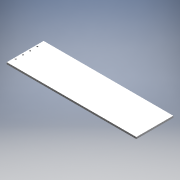
# Autodesk Inventor part: AluminumPlateForWinch
Saved by Autodesk Inventor 2018.2 (Build 222227000, 227)
## iProperties
Created: 2018-01-31
Part Number: AluminumPlateForWinch
Material: Aluminum 6061
Document SubType Name: Modeling
Designer: steele
Mass: 1020.4 g
Surface Area: 1264.92 cm^2
Volume: 377.927 cm^3
Density: 2.7 g/cm^3
Appearance: Aluminum - Flat
Author: steele
Autodesk Inventor part; units mm, degrees
ref_plane "YZ Plane" through (0, 0, 0) normal (1, 0, 0) x (0, 1, 0)
ref_plane "XZ Plane" through (0, 0, 0) normal (0, 1, 0) x (-1, 0, 0)
ref_plane "XY Plane" through (0, 0, 0) normal (0, 0, 1) x (1, 0, 0)
sketch "Sketch1" plane through (0, 0, 0) normal (0, 1, 0) x (-1, 0, 0)
  line L0 (228.6, 65.0875) -> (-228.6, 65.0875)
  line L1 (-228.6, 65.0875) -> (-228.6, -65.0875)
  line L2 (-228.6, -65.0875) -> (228.6, -65.0875)
  line L3 (228.6, -65.0875) -> (228.6, 65.0875)
  line L4 (228.6, 65.0875) -> (-228.6, -65.0875) construction
  line L5 (-228.6, 65.0875) -> (228.6, -65.0875) construction
  point P0 (0, 0)
  dimension "d0" = 457.2
  dimension "d1" = 130.175
  constraints: 12 end point, 2 midpoint, 2 parallel, 1 horizontal, 1 perpendicular
  measures "d0" distance of L0.start L0.end
  measures "d1" distance of L1.end L0.end
extrude "Extrusion1" add sketch "Sketch1" along normal blind 6.35
sketch "Sketch2" plane through (0, 6.35, 0) normal (0, 1, 0) x (1, 0, 0)
  line L0 (-228.6, -65.0875) -> (228.6, -65.0875) construction
  line L1 (-222.25, -65.0875) -> (-222.25, 65.0875) construction
  line L2 (228.6, 65.0875) -> (-228.6, 65.0875) construction
  line L3 (-228.6, 65.0875) -> (-228.6, -65.0875) projected
  point P0 (0, 0)
  point P1 (-222.25, -39.6875)
  point P2 (-222.25, -14.2875)
  point P3 (-222.25, 11.1125)
  point P4 (-222.25, 36.5125)
  dimension "d4" = 6.35
  dimension "d5" = 25.4
  dimension "d8" = 25.4
  constraints: 3 point on line, 2 end point, 2 vertical, 3 other
  measures "d4" distance between parallel lines of L1 L3
  measures "d5" distance from line of L0 point (-222.25, -39.688)
  measures "d8" distance of point (-222.25, -39.688) point (-222.25, -14.288)
hole "Hole1" at (-222.25, 6.35, 39.6875) at (-222.25, 6.35, 14.2875) at (-222.25, 6.35, -11.1125) at (-222.25, 6.35, -36.5125) direction (0, -1, 0) diameter 5.1054 end through all clearance for "Flat Head Machine Screw (82)" size "#10" standard "Ansi Unified Screw Threads"
mirror "Mirror1" about plane through (0, 0, 0) normal (1, 0, 0) of "Hole1"
body "Solid1"
